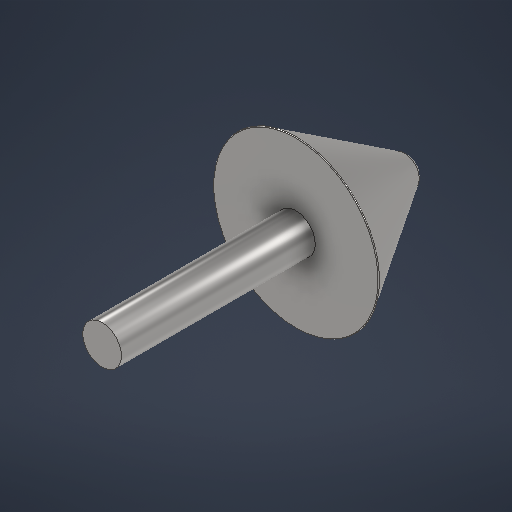
# Autodesk Inventor part: ConoEntrata
Saved by Autodesk Inventor 2026.2 (Build 302298010, 298A)
## iProperties
Created: 2026-05-01
Part Number: ConoEntrata
Material: Steel, Alloy
Document SubType Name: Modeling
Designer: Yan
Density: 7.73 g/cm^3
Appearance: Semi-Polished
Author: Yan
Autodesk Inventor part; units mm, degrees
ref_plane "YZ Plane" through (0, 0, 0) normal (1, 0, 0) x (0, 1, 0)
ref_plane "XZ Plane" through (0, 0, 0) normal (0, 1, 0) x (-1, 0, 0)
ref_plane "XY Plane" through (0, 0, 0) normal (0, 0, 1) x (1, 0, 0)
sketch "Sketch1" plane through (0, 0, 0) normal (1, 0, 0) x (0, 1, 0)
  line L0 (0, 0) -> (0, -540)
  line L1 (0, 0) -> (34, 0)
  line L2 (34, 0) -> (34, -340)
  line L3 (34, -340) -> (146, -340)
  line L4 (0, -540) -> (20, -540)
  line L5 (20, -540) -> (146, -340)
  dimension "d0" = 68
  dimension "d1" = 112
  dimension "d2" = 20
  dimension "d3" = 540
  dimension "d4" = 340
  constraints: 12 end point, 2 horizontal, 2 perpendicular, 1 vertical
  measures "d0" diameter of L2 L0
  measures "d1" distance of L2.end L3.end
  measures "d2" distance of L0.end L4.end
  measures "d3" distance of L0.start L0.end
  measures "d4" distance of L1.end L2.end
revolve "Revolution1" add sketch "Sketch1" angle 360 about axis through (0, 0, 0) along (0, 0, -1)
fillet "Fillet1" radius 20 1 edges at (0, -20, -540)
fillet "Fillet2" radius 1 1 edges at (0, -146, -340)
body "Solid1"
